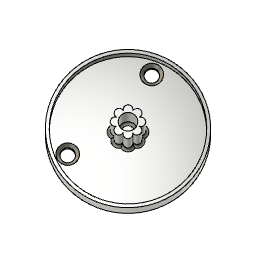
KitchenBlindSupport v6 (Autodesk Fusion 360 design; units mm, degrees)
Autodesk Fusion 360 part; units mm, degrees
note: some values were not read from the file. Set by a fixed rule: which sketch regions a step uses.
sketch "Sketch1" plane through (0, 0, 0) normal (0, 0, 1) x (1, 0, 0) in component "BlindSupport"
  circle A0 centre (0, 0) radius 20
  circle A1 centre (0, 0) radius 21
  circle A2 centre (0, 0) radius 2.5
  circle A3 centre (0, 0) radius 4.5
  line L0 (0, 0) -> (0, 4.5)
  line L1 (0, 0) -> (-3.182, 3.182)
  line L2 (0, 0) -> (-4.5, 0)
  line L3 (0, 0) -> (-3.182, -3.182)
  line L4 (0, 0) -> (0, -4.5)
  line L5 (0, 0) -> (3.182, -3.182)
  line L6 (0, 0) -> (4.5, 0)
  line L7 (0, 0) -> (3.182, 3.182)
  line L8 (0, 0) -> (0, 40.0695) construction
  circle A4 centre (-15, 6.5991) radius 2
  circle A5 centre (15, 6.5991) radius 2
  line L9 (15, 6.5991) -> (-15, 6.5991) construction
  line L10 (-19.5984, 22.5991) -> (25.099, 22.5991) construction
  circle A6 centre (0, 3.25) radius 1.25
  circle A7 centre (-2.2981, 2.2981) radius 1.25
  circle A8 centre (-3.25, 0) radius 1.25
  circle A9 centre (-2.2981, -2.2981) radius 1.25
  circle A10 centre (0, -3.25) radius 1.25
  circle A11 centre (2.2981, -2.2981) radius 1.25
  circle A12 centre (3.25, 0) radius 1.25
  circle A13 centre (2.2981, 2.2981) radius 1.25
  point P0 (0, 6.5991)
  point P1 (-15, 6.5991)
  dimension "d1" = 40
  dimension "d2" = 1
  dimension "d3" = 5
  dimension "d4" = 9
  dimension "d6" = 360
  dimension "d7" = 4
  dimension "d8" = 30
  dimension "d9" = 16
  dimension "d12" = 2.5
  dimension "d14" = 360
  constraint coincident A0.centre A1.centre
  constraint concentric A0 A2
  constraint concentric A0 A3
  constraint coincident A3 L0.end
  constraint vertical L0
  constraint perpendicular L2 L8
  constraint equal A4 A5
  constraint coincident A5.centre L9
  constraint coincident P1 L9
  constraint horizontal L9
  constraint coincident A5.centre L9.start
  constraint coincident P1 A4.centre
  constraint midpoint L9 P0
  constraint coincident L8 P0
  constraint horizontal L10
  constraint coincident L0.end A6
  constraint tangent A3 A6
  measures "d1" diameter of A0
  measures "d3" diameter of A2
  measures "d4" diameter of A3
  measures "d7" diameter of A4
  measures "d8" distance of P1 A5.centre
  measures "d9" distance of L9 L10
  measures "d12" diameter of A6
extrude "Extrude1" add sketch "Sketch1" along normal blind 2 contours A0 | A1 | A2 L6 A12 | A2 L6 A11 A12 | A2 L6 A12 A13 | A2 L6 A12 | A2 L6 L7 A12 A13 | A2 A12 A13 | A2 A11 A12 | A2 L5 L6 A11 A12 | A3 A12 A13 | A3 A11 A12 | A2 L7 A13 | A2 L7 A12 A13 | A12 A13 | A2 L5 A11 A12 | A2 L5 A11 | A11 A12 | A3 A6 A13 | A2 L7 A6 A13 | A2 L5 A10 A11 | A3 A10 A11 | A2 L0 L1 A6 A7 | A2 L1 L2 A7 A8 | A2 L2 L3 A8 A9 | A2 L3 L4 A9 A10 | A2 L4 L5 A10 A11 | A2 L0 L7 A6 A13 | A2 L7 A13 | A2 L5 A11 | A3 A6 A7 | A2 L0 A6 A13 | A2 L0 A6 A7 | A6 A13 | A2 L4 A9 A10 | A2 L4 A10 A11 | A3 A9 A10 | A10 A11 | A2 L0 A6 | A2 L0 A6 | A2 L1 A7 | A2 L1 A7 | A2 L2 A8 | A2 L2 A8 | A2 L3 A9 | A2 L3 A9 | A2 L4 A10 | A2 L4 A10 | A2 A6 A13 | A2 A10 A11 | A3 A7 A8 | A2 L1 A6 A7 | A2 L1 A7 A8 | A6 A7 | A2 L3 A8 A9 | A3 A8 A9 | A2 L3 A9 A10 | A9 A10 | A2 A6 A7 | A2 A7 A8 | A2 L2 A7 A8 | A2 L2 A8 A9 | A2 A8 A9 | A2 A9 A10 | A7 A8 | A8 A9 | A4 | A5 in component "BlindSupport"
extrude "Extrude2" add sketch "Sketch1" against normal blind 9 contours A2 L6 A11 A12 | A2 L6 A12 A13 | A2 A12 A13 | A2 A11 A12 | A2 L7 A12 A13 | A12 A13 | A2 L5 A11 A12 | A11 A12 | A2 L7 A6 A13 | A2 L5 A10 A11 | A2 L0 A6 A13 | A2 L0 A6 A7 | A6 A13 | A2 L4 A9 A10 | A2 L4 A10 A11 | A10 A11 | A2 A6 A13 | A2 A10 A11 | A2 L1 A6 A7 | A2 L1 A7 A8 | A6 A7 | A2 L3 A8 A9 | A2 L3 A9 A10 | A9 A10 | A2 A6 A7 | A2 A7 A8 | A2 L2 A7 A8 | A2 L2 A8 A9 | A2 A8 A9 | A2 A9 A10 | A7 A8 | A8 A9 in component "BlindSupport"
extrude "Extrude3" add sketch "Sketch1" against normal blind 3 contours A1 in component "BlindSupport"
sketch "Sketch2" plane through (0, 0, 2) normal (0, 0, 1) x (-1, 0, 0) in component "BlindSupport"
  circle A0 centre (0, 0) radius 21
  point P0 (-15, -6.5991)
  point P1 (15, -6.5991)
hole "Hole1" at (-15.02, 6.591, 0) direction (0, 0, 1) diameter 4 depth 4.5 tip angle 118 countersink diameter 6 countersink angle 90 in component "BlindSupport"
mirror "Mirror1" about plane through (0, 0, 0) normal (1, 0, 0) of "Hole1" in component "BlindSupport"
fillet "Fillet1" radius 0.8 8 edges at (0, -4.5, 0) (3.182, -3.182, 0) (4.5, 0, 0) (3.182, 3.182, 0) (0, 4.5, 0) (-3.182, 3.182, 0) (-4.5, 0, 0) (-3.182, -3.182, 0) in component "BlindSupport"
fillet "Fillet2" radius 0.8 1 edges at (-2.3308, 0.904, 0) in component "BlindSupport"
component "BlindSupport" placed x (1, 0, 0) y (0, 1, 0) z (0, 0, 1) at (0, 0, 0)
named bodies: "kitchenBlindSupport"
